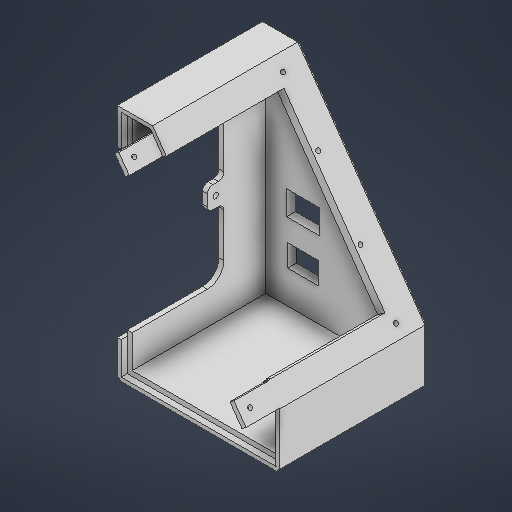
# Autodesk Inventor part: case3
Saved by Autodesk Inventor 2026.2 (Build 302298000, 298)
## iProperties
Created: 2026-01-28
Part Number: case3
Material: Generic
Document SubType Name: Modeling
Designer: test
Density: 1 g/cm^3
Appearance: Default
Author: test
## iProperties of the stored document case4_3DPrint.ipt
Created: 2026-01-28
Part Number: case4_3DPrint
Material: Generic
Document SubType Name: Modeling
Designer: test
Density: 1 g/cm^3
Appearance: Default
Author: test
Autodesk Inventor part; units mm, degrees
ref_plane "YZ Plane" through (0, 0, 0) normal (1, 0, 0) x (0, 1, 0)
ref_plane "XZ Plane" through (0, 0, 0) normal (0, 1, 0) x (-1, 0, 0)
ref_plane "XY Plane" through (0, 0, 0) normal (0, 0, 1) x (1, 0, 0)
sketch "Sketch1" plane through (0, 0, 0) normal (0, 0, 1) x (1, 0, 0)
  line L0 (0, 0) -> (0, 199.7346)
  line L1 (0, 199.7346) -> (20, 199.7346)
  line L2 (20, 199.7346) -> (131.8474, 40)
  line L3 (131.8474, 40) -> (131.8474, 0)
  line L4 (131.8474, 0) -> (0, 0)
  dimension "d0" = 40
  dimension "d1" = 55
  dimension "d2" = 20
  dimension "d3" = 195
  constraints: 10 end point, 2 perpendicular, 1 parallel, 1 vertical
  measures "d0" distance of L2.end L3.end
  measures "d1" angle of L4 L2
  measures "d2" distance of L0.end L1.end
  measures "d3" distance of L1.end L2.end
extrude "Extrusion1" add sketch "Sketch1" along normal blind 127.11
sketch "Sketch5" plane through (131.8474, 40, 0) normal (0.819152, 0.5735764, 0) x (0, 0, -1)
  line L0 (-127.11, 206.4715) -> (-127.11, 42.8585) projected
  line L1 (-127.11, 177.5) -> (-20, 177.5)
  line L2 (-20, 177.5) -> (-20, 17.5)
  line L3 (-20, 17.5) -> (-127.11, 17.5)
  line L4 (-127.11, 17.5) -> (-127.11, 177.5)
  line L5 (0, 0) -> (0, 195) projected
  line L6 (0, 195) -> (-127.11, 195) projected
  line L7 (0, 0) -> (-127.11, 0) projected
  line L8 (0, 97.5) -> (-127.11, 97.5) construction
  point P0 (0, 42.8585)
  point P1 (-127.11, 42.8585)
  point P2 (-20, 97.5)
  dimension "d33" = 160
  dimension "d57" = 20
  constraints: 10 end point, 3 midpoint, 2 parallel, 2 point on line, 1 horizontal, 1 perpendicular
  measures "d33" distance between parallel lines of L3 L1
  measures "d57" distance between parallel lines of L5 L2
extrude "Extrusion5" cut sketch "Sketch5" against normal blind 10
shell "Shell2" thickness 8 outward yes removed faces 5 at (45.1537, 76.0869, 127.11) at (83.0259, 92.2864, 55.7033) at (119.0788, 52.4229, 91.4067) at (27.3065, 183.4872, 55.7033) at (55.1662, 137.8868, 20)
sketch "Sketch3" plane through (20, 199.7346, 0) normal (0.819152, 0.5735764, 0) x (0, 0, -1)
  line L0 (-127.11, -197.5224) -> (-127.11, -177.5) projected
  line L1 (8, 4.1645) -> (-127.11, 4.1645) projected
  line L2 (8, -197.5224) -> (8, 4.1645) projected
  line L3 (8, -197.5224) -> (-127.11, -197.5224) projected
  line L4 (-127.11, -17.5) -> (-127.11, 4.1645) projected
  line L5 (-189.4203, -97.5) -> (-20, -97.5) construction
  circle A0 centre (-15.5, -64) radius 2
  circle A1 centre (-15.5, -8) radius 2
  circle A2 centre (-15.5, -131) radius 2
  circle A3 centre (-15.5, -187) radius 2
  line L6 (-15.5, 86.5068) -> (-15.5, -64) construction
  line L7 (-20, -177.5) -> (-127.11, -177.5) projected
  line L8 (-20, -17.5) -> (-20, -177.5) projected
  line L9 (-127.11, -17.5) -> (-20, -17.5) projected
  line L10 (-15.5, -187) -> (-15.5, -8) construction
  line L11 (0, -195) -> (-127.11, -195) projected
  line L12 (-20, -17.5) -> (-20, -177.5) projected
  point P0 (0, -152.1415)
  point P1 (10, -200.2057)
  dimension "d22" = 4
  dimension "d23" = 4
  dimension "d24" = 4
  dimension "d25" = 4
  dimension "d35" = 179
  dimension "d43" = 67
  dimension "d58" = 4.5
  constraints: 6 end point, 4 centre point, 3 point on line, 2 symmetric about line, 1 coincident, 1 midpoint, 1 vertical, 1 other
  measures "d22" diameter of A3
  measures "d23" diameter of A2
  measures "d24" diameter of A0
  measures "d25" diameter of A1
  measures "d35" distance of A3.centre L10.end
  measures "d43" distance of A2.centre L6.end
  measures "d58" distance between parallel lines of L8 L10
extrude "Extrusion4" cut sketch "Sketch3" along normal up to surface (8 mm away) contours A0 | A1 | A2 | A3
sketch "Sketch6" plane through (0, 0, 127.11) normal (0, 0, 1) x (-1, 0, 0)
  line L0 (-20, -199.7346) -> (-30.0376, -185.3995) projected
  line L1 (0, -199.7346) -> (-20, -199.7346) projected
  line L2 (0, 0) -> (0, -199.7346) projected
  line L3 (-131.8474, 0) -> (0, 0) projected
  line L4 (-131.8474, -40) -> (-131.8474, 0) projected
  line L5 (-121.8098, -54.3352) -> (-131.8474, -40) projected
  line L6 (-128.363, -58.9238) -> (-121.8098, -54.3352) projected
  line L7 (-36.5908, -189.9881) -> (-24.1645, -207.7346) projected
  line L8 (-139.8474, 8) -> (-139.8474, -42.5224) projected
  line L9 (8, 8) -> (-139.8474, 8) projected
  line L10 (8, -207.7346) -> (8, 8) projected
  line L11 (-24.1645, -207.7346) -> (8, -207.7346) projected
  line L12 (-139.8474, -42.5224) -> (-128.363, -58.9238) projected
  line L13 (-30.0376, -185.3995) -> (-36.5908, -189.9881) projected
  line L14 (-22.3426, -204.2346) -> (-33.7238, -187.9806)
  line L15 (-125.496, -56.9163) -> (-136.3474, -41.4188)
  line L16 (-136.3474, -41.4188) -> (-136.3474, 4.5)
  line L17 (4.5, 4.5) -> (4.5, -204.2346)
  line L18 (4.5, -204.2346) -> (-22.3426, -204.2346)
  line L19 (4.5, 4.5) -> (-136.3474, 4.5)
  dimension "d59" = 3.5
  dimension "d60" = 3.5
  dimension "d106" = 3.5
  dimension "d107" = 3.5
  dimension "d108" = 3.5
  constraints: 12 end point, 2 parallel, 2 point on line, 1 vertical, 1 other
  measures "d59" distance between parallel lines of L7 L14
  measures "d60" distance between parallel lines of L11 L18
  measures "d106" distance between parallel lines of L10 L17
  measures "d107" distance between parallel lines of L9 L19
  measures "d108" distance between parallel lines of L8 L16
extrude "Extrusion6" cut sketch "Sketch6" against normal blind 5.5 contours L1 L2 L3 L4 L5 L6 L15 L16 L19 L17 L18 L14 L13 L0
sketch "Sketch10" plane through (139.8474, 42.5224, 127.11) normal (0.819152, 0.5735764, 0) x (0, 0, -1)
  circle A0 centre (111.61, 133.5224) radius 2 projected
  circle A1 centre (111.61, 66.5224) radius 2 projected
  circle A2 centre (111.61, 189.5224) radius 2 projected
  circle A3 centre (111.61, 10.5224) radius 2 projected
  line L0 (107.11, 20.0224) -> (0, 20.0224) projected
  line L1 (0, 0) -> (0, 20.0224) projected
  line L2 (135.11, 0) -> (0, 0) projected
  line L3 (135.11, 0) -> (135.11, 201.6869) projected
  line L4 (135.11, 201.6869) -> (0, 201.6869) projected
  line L5 (0, 180.0224) -> (0, 201.6869) projected
  line L6 (0, 180.0224) -> (107.11, 180.0224) projected
  line L7 (107.11, 180.0224) -> (107.11, 20.0224) projected
  line L8 (135.11, 0) -> (0, 0) projected
  line L9 (0, 0) -> (-30.945, 0)
  line L10 (-30.945, 0) -> (-30.945, 20.0224)
  line L11 (-30.945, 20.0224) -> (0, 20.0224)
  line L12 (0, 20.0224) -> (0, 0)
  circle A4 centre (-20.945, 10.5224) radius 2
  line L13 (-20.945, 10.5224) -> (111.61, 10.5224) construction
  line L14 (-0.5, 19.5224) -> (-30.445, 19.5224)
  line L15 (-30.445, 19.5224) -> (-30.445, 0.5)
  line L16 (-30.445, 0.5) -> (-0.5, 0.5)
  line L17 (-0.5, 0.5) -> (-0.5, 19.5224)
  line L18 (-0.5, 19.5224) -> (0, 19.5224)
  line L19 (0, 19.5224) -> (0, 0.5)
  line L20 (0, 0.5) -> (-0.5, 0.5)
  line L21 (-0.5, 0.5) -> (-0.5, 19.5224)
  line L22 (5.5, 199.8649) -> (5.5, 180.0224) projected
  line L23 (5.5, 215.2612) -> (5.5, 199.8649) projected
  line L24 (5.5, 44.2758) -> (5.5, 215.2612) projected
  line L25 (5.5, -36.511) -> (5.5, 44.2758) projected
  line L26 (5.5, 1.1035) -> (5.5, -36.511) projected
  line L27 (5.5, 20.0224) -> (5.5, 1.1035) projected
  line L28 (5.5, 2.5224) -> (5.5, 20.0224) projected
  line L29 (5.5, -30.2437) -> (5.5, 2.5224) projected
  line L30 (5.5, 45.3809) -> (5.5, -30.2437) projected
  line L31 (5.5, 208.9939) -> (5.5, 45.3809) projected
  line L32 (5.5, 197.5224) -> (5.5, 208.9939) projected
  line L33 (5.5, 180.0224) -> (5.5, 197.5224) projected
  point P0 (127.11, 45.3809)
  point P1 (0, 0.5)
  point P2 (0, 19.5224)
  point P3 (5.5, 0)
  dimension "d67" = 4
  dimension "d68" = 132.555
  dimension "d69" = 10
  dimension "d70" = 0.5
  constraints: 26 end point, 7 parallel, 3 perpendicular, 2 horizontal, 2 point on line, 1 centre point, 3 other
  measures "d67" diameter of A4
  measures "d68" distance of L13.end L13.start
  measures "d69" distance from line of L13.start L10
  measures "d70" distance between parallel lines of L11 L14
extrude "Extrusion10" add sketch "Sketch10" against normal blind 4.5 contours L25 L2 L1 L0 | L1 L20 L17 L18 | L17 L16 L15 L14
sketch "Sketch11" plane through (20, 199.7346, 0) normal (-0.819152, -0.5735764, 0) x (0, 0, 1)
  line L0 (121.61, -195) -> (121.61, -177.5) projected
  line L1 (20, -177.5) -> (121.61, -177.5) projected
  line L2 (20, -17.5) -> (20, -177.5) projected
  line L3 (121.61, -17.5) -> (20, -17.5) projected
  line L4 (121.61, -17.5) -> (121.61, 0) projected
  line L5 (0, 0) -> (121.61, 0) projected
  line L6 (0, -195) -> (0, 0) projected
  line L7 (0, -195) -> (121.61, -195) projected
  circle A0 centre (15.5, -64) radius 2 projected
  circle A1 centre (15.5, -131) radius 2 projected
  circle A2 centre (15.5, -8) radius 2 projected
  circle A3 centre (15.5, -187) radius 2 projected
  line L8 (121.61, -17.5) -> (158.055, -17.5)
  line L9 (158.055, -17.5) -> (158.055, 0)
  line L10 (158.055, 0) -> (121.61, 0)
  line L11 (121.61, 0) -> (121.61, -17.5)
  circle A4 centre (148.055, -8) radius 2
  line L12 (15.5, -8) -> (148.055, -8) construction
  line L13 (122.11, -0.5) -> (157.555, -0.5)
  line L14 (157.555, -0.5) -> (157.555, -17)
  line L15 (157.555, -17) -> (122.11, -17)
  line L16 (122.11, -17) -> (122.11, -0.5)
  line L17 (122.11, -0.5) -> (121.61, -0.5)
  line L18 (121.61, -0.5) -> (121.61, -17)
  line L19 (121.61, -17) -> (122.11, -17)
  line L20 (122.11, -17) -> (122.11, -0.5)
  point P0 (0, -152.1415)
  point P1 (121.61, -0.5)
  point P2 (121.61, -17)
  dimension "d73" = 4
  dimension "d74" = 132.555
  dimension "d75" = 10
  dimension "d76" = 0.5
  constraints: 26 end point, 7 parallel, 3 horizontal, 3 perpendicular, 1 centre point, 1 point on line, 3 other
  measures "d73" diameter of A4
  measures "d74" distance of L12.start L12.end
  measures "d75" distance from line of L9 L12.end
  measures "d76" distance between parallel lines of L10 L13
extrude "Extrusion11" add sketch "Sketch11" against normal blind 4.5 contours L17 L16 L19 L4 | L13 L14 L15 L16
sketch "Sketch12" plane through (-8, -8, -8) normal (-1, 0, 0) x (0, 0, 1)
  line L0 (61.055, 182.8673) -> (271.055, 182.8673)
  line L1 (291.055, 162.8673) -> (291.055, 52.8673)
  line L2 (271.055, 32.8673) -> (61.055, 32.8673)
  line L3 (41.055, 52.8673) -> (41.055, 162.8673)
  arc A0 (41.055, 52.8673) -> (61.055, 32.8673) centre (61.055, 52.8673) ccw
  arc A1 (61.055, 182.8673) -> (41.055, 162.8673) centre (61.055, 162.8673) ccw
  arc A2 (291.055, 162.8673) -> (271.055, 182.8673) centre (271.055, 162.8673) ccw
  arc A3 (271.055, 32.8673) -> (291.055, 52.8673) centre (271.055, 52.8673) ccw
  line L4 (0, 215.7346) -> (0, 0) projected
  line L5 (0, 107.8673) -> (41.055, 107.8673) construction
  point P0 (8, 8)
  point P1 (166.055, 32.8673)
  dimension "d79" = 150
  dimension "d80" = 250
  dimension "d81" = 20
  dimension "d82" = 166.055
  constraints: 10 end point, 8 point on circle, 8 tangent, 4 centre point, 3 equal radius, 3 midpoint, 2 parallel, 2 perpendicular, 1 horizontal
  measures "d79" distance between parallel lines of L2 L0
  measures "d80" distance between parallel lines of L1 L3
  measures "d81" radius of A0
  measures "d82" distance from line of L4 point (166.055, 32.867)
extrude "Extrusion12" cut sketch "Sketch12" against normal blind 3.5
sketch "Sketch13" plane through (-4.5, -8, -8) normal (-1, 0, 0) x (0, 0, 1)
  line L0 (129.61, 32.8673) -> (129.61, 182.8673) projected
  line L1 (61.055, 182.8673) -> (129.61, 182.8673) projected
  arc A0 (61.055, 182.8673) -> (41.055, 162.8673) centre (61.055, 162.8673) ccw projected
  line L2 (41.055, 52.8673) -> (41.055, 162.8673) projected
  arc A1 (41.055, 52.8673) -> (61.055, 32.8673) centre (61.055, 52.8673) ccw projected
  line L3 (129.61, 32.8673) -> (61.055, 32.8673) projected
  line L4 (124.61, 177.8673) -> (124.61, 37.8673)
  line L5 (124.61, 37.8673) -> (61.055, 37.8673)
  arc A2 (46.055, 52.8673) -> (61.055, 37.8673) centre (61.055, 52.8673) ccw
  line L6 (46.055, 52.8673) -> (46.055, 162.8673)
  arc A3 (61.055, 177.8673) -> (46.055, 162.8673) centre (61.055, 162.8673) ccw
  line L7 (61.055, 177.8673) -> (124.61, 177.8673)
  line L8 (124.61, 177.8673) -> (129.61, 177.8673)
  line L9 (129.61, 177.8673) -> (129.61, 37.8673)
  line L10 (129.61, 37.8673) -> (124.61, 37.8673)
  line L11 (124.61, 37.8673) -> (124.61, 177.8673)
  line L12 (46.055, 117.8673) -> (61.055, 117.8673)
  line L13 (61.055, 117.8673) -> (61.055, 97.8673)
  line L14 (61.055, 97.8673) -> (46.055, 97.8673)
  line L15 (46.055, 97.8673) -> (46.055, 117.8673)
  circle A4 centre (53.555, 107.8673) radius 2.5
  line L16 (61.055, 97.8673) -> (53.555, 97.8673) construction
  line L17 (53.555, 97.8673) -> (53.555, 107.8673) construction
  line L18 (53.555, 107.8673) -> (61.055, 107.8673) construction
  line L19 (61.055, 107.8673) -> (61.055, 97.8673) construction
  point P0 (8, 8)
  point P1 (46.055, 107.8673)
  dimension "d85" = 5
  dimension "d88" = 20
  dimension "d89" = 20
  dimension "d90" = 5
  dimension "d91" = 7.5
  dimension "d92" = 10
  constraints: 32 end point, 6 parallel, 4 point on circle, 3 centre point, 3 horizontal, 3 perpendicular, 2 midpoint, 2 point on line, 5 other
  measures "d85" distance between parallel lines of L1 L7
  measures "d88" distance between parallel lines of L14 L12
  measures "d89" distance between parallel lines of L2 L13
  measures "d90" diameter of A4
  measures "d91" distance between parallel lines of L19 L17
  measures "d92" distance between parallel lines of L16 L18
extrude "Extrusion13" cut sketch "Sketch13" against normal up to surface (4.5 mm away) contours L10 L4 L8 L0 | L5 A2 L6 L14 L13 L12 A3 L7 L4 | A4
chamfer "Chamfer1" distance 3 angle 45 7 edges at (82.006, 125.1285, -8) (139.8474, 17.2612, -8) (65.9237, -8, -8) (-8, 99.8673, -8) (8.0823, 207.7346, -8) (139.8474, -8, 59.555) (-8, -8, 59.555)
fillet "Fillet2" radius 5 4 edges at (-2.25, 109.8673, 53.055) (-2.25, 89.8673, 53.055) (-2.25, 109.8673, 38.055) (-2.25, 89.8673, 38.055)
sketch "Sketch14" plane through (0, 0, -8) normal (0, 0, -1) x (-1, 0, 0)
  line L0 (-49, 92) -> (-19, 92)
  line L1 (-19, 92) -> (-19, 70)
  line L2 (-19, 70) -> (-49, 70)
  line L3 (-49, 70) -> (-49, 92)
  line L4 (-48, 50) -> (-20, 50)
  line L5 (-20, 50) -> (-20, 30)
  line L6 (-20, 30) -> (-48, 30)
  line L7 (-48, 30) -> (-48, 50)
  line L8 (0, 0) -> (-131.8474, 0) projected
  line L9 (0, 0) -> (-131.8474, 0) projected
  line L10 (0, 89.8673) -> (0, 94.8673) projected
  line L11 (0, 84.8673) -> (0, 89.8673) projected
  line L12 (0, 84.8673) -> (0, 44.8673) projected
  line L13 (0, 44.8673) -> (0, 29.8673) projected
  line L14 (0, 29.8673) -> (0, 0) projected
  line L15 (0, 199.7346) -> (0, 0) projected
  line L16 (0, 199.7346) -> (0, 169.8673) projected
  line L17 (0, 169.8673) -> (0, 154.8673) projected
  line L18 (0, 154.8673) -> (0, 114.8673) projected
  line L19 (0, 109.8673) -> (0, 114.8673) projected
  line L20 (0, 104.8673) -> (0, 109.8673) projected
  line L21 (0, 104.8673) -> (0, 94.8673) projected
  line L22 (0, 97.3673) -> (0, 102.3673) projected
  line L23 (-34, 50) -> (-34, 70) construction
  dimension "d99" = 20
  dimension "d100" = 28
  dimension "d101" = 20
  dimension "d102" = 30
  dimension "d103" = 22
  dimension "d104" = 30
  dimension "d105" = 20
  constraints: 18 end point, 4 parallel, 3 perpendicular, 2 horizontal, 2 midpoint
  measures "d99" distance between parallel lines of L6 L4
  measures "d100" distance between parallel lines of L5 L7
  measures "d101" distance between parallel lines of L14 L5
  measures "d102" distance between parallel lines of L8 L6
  measures "d103" distance between parallel lines of L0 L2
  measures "d104" distance between parallel lines of L3 L1
  measures "d105" distance between parallel lines of L2 L4
extrude "Extrusion14" cut sketch "Sketch14" against normal up to surface (8 mm away)
equation "\"d23\" = d22"
body "Solid1"
